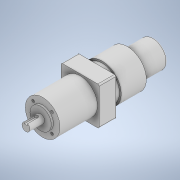
# Autodesk Inventor part: Motor
Saved by Autodesk Inventor 2020 (Build 240168000, 168)
## iProperties
Created: 2022-06-08
Part Number: Motor
Material: 일반
Document SubType Name: Modeling
Designer: samsung
Density: 1 g/cm^3
Appearance: 기본값
Mass: 368.156 g
Surface Area: 370.371 cm^2
Volume: 368.156 cm^3
Author: samsung
Autodesk Inventor part; units mm, degrees
ref_plane "YZ Plane" through (0, 0, 0) normal (1, 0, 0) x (0, 1, 0)
ref_plane "XZ Plane" through (0, 0, 0) normal (0, 1, 0) x (-1, 0, 0)
ref_plane "XY Plane" through (0, 0, 0) normal (0, 0, 1) x (1, 0, 0)
sketch "스케치1" plane through (0, 0, 0) normal (0, 0, 1) x (1, 0, 0)
  line L0 (-26.5, -28.5) -> (26.5, -28.5)
  line L1 (28.5, -26.5) -> (28.5, 26.5)
  line L2 (26.5, 28.5) -> (-26.5, 28.5)
  line L3 (-28.5, 26.5) -> (-28.5, -26.5)
  line L4 (-28.5, -28.5) -> (28.5, 28.5) construction
  line L5 (28.5, -28.5) -> (-28.5, 28.5) construction
  arc A0 (28.5, 26.5) -> (26.5, 28.5) centre (26.5, 26.5) ccw
  arc A1 (26.5, -28.5) -> (28.5, -26.5) centre (26.5, -26.5) ccw
  arc A2 (-28.5, -26.5) -> (-26.5, -28.5) centre (-26.5, -26.5) ccw
  arc A3 (-26.5, 28.5) -> (-28.5, 26.5) centre (-26.5, 26.5) ccw
  point P0 (0, 0)
  dimension "d0" = 57
  dimension "d1" = 57
  dimension "d2" = 2
  constraints: 12 end point, 8 point on circle, 8 point on line, 8 tangent, 4 centre point, 3 equal radius, 2 midpoint, 2 parallel, 1 horizontal, 1 perpendicular
  measures "d0" distance of L5.end L4.end
  measures "d1" distance of L4.end L5.start
  measures "d2" radius of A0
extrude "돌출1" add sketch "스케치1" along normal blind 25
sketch "스케치2" plane through (0, 0, 25) normal (0, 0, 1) x (1, 0, 0)
  circle A0 centre (0, 0) radius 26
  dimension "d5" = 52
  constraints: 1 centre point, 1 coincident
  measures "d5" diameter of A0
extrude "돌출2" add sketch "스케치2" along normal blind 56.1
sketch "스케치3" plane through (0, 0, 81.1) normal (0, 0, 1) x (1, 0, 0)
  circle A0 centre (0, 0) radius 16
  line L0 (0, 0) -> (20, 0) construction
  circle A1 centre (0, 0) radius 15
  point P0 (-14.1421, 14.1421)
  point P1 (-14.1421, -14.1421)
  point P2 (14.1421, -14.1421)
  point P3 (14.1421, 14.1421)
  dimension "d9" = 32
  dimension "d16" = 30
  constraints: 2 centre point, 2 end point, 1 coincident, 1 horizontal
  measures "d9" diameter of A0
  measures "d16" diameter of A1
sketch "스케치4" plane through (0, 0, 81.1) normal (0, 0, 1) x (1, 0, 0)
  circle A0 centre (0, 0) radius 16
  dimension "d21" = 32
  constraints: 1 centre point, 1 coincident
  measures "d21" diameter of A0
extrude "돌출5" add sketch "스케치4" along normal blind 3
sketch "스케치5" plane through (0, 0, 84.1) normal (0, 0, 1) x (1, 0, 0)
  circle A0 centre (0, 0) radius 6
  dimension "d24" = 12
  constraints: 1 centre point, 1 coincident
  measures "d24" diameter of A0
extrude "돌출6" add sketch "스케치5" along normal blind 22
sketch "스케치6" plane through (0, 0, 106.1) normal (0, 0, 1) x (1, 0, 0)
  circle A0 centre (0, 0) radius 6 projected
  circle A1 centre (0, 0) radius 6 projected
  line L0 (-2.5, 5.4544) -> (2.5, 5.4544)
  line L1 (2.5, 5.4544) -> (2.5, 2.9544)
  line L2 (2.5, 2.9544) -> (-2.5, 2.9544)
  line L3 (-2.5, 2.9544) -> (-2.5, 5.4544)
  line L4 (-2.5, 5.4544) -> (2.5, 5.4544)
  line L5 (2.5, 5.4544) -> (2.5, 6.5478)
  line L6 (2.5, 6.5478) -> (-2.5, 6.5478)
  line L7 (-2.5, 6.5478) -> (-2.5, 5.4544)
  dimension "d29" = 2.5
  constraints: 16 end point, 4 parallel, 2 horizontal, 2 perpendicular, 2 other
  measures "d29" distance of L0.end L1.end
extrude "돌출7" cut sketch "스케치6" against normal blind 15.5 contours L0 A0 | L1 L2 L3 L0 | A0 L7 L6 L5
sketch "스케치7" plane through (-2.5, 2.9544, 106.1) normal (0, 1, 0) x (1, 0, 0)
  line L0 (5, 0) -> (0, 0) projected
  line L1 (5, 0) -> (5, 15.5) projected
  line L2 (5, 15.5) -> (0, 15.5) projected
  line L3 (0, 0) -> (0, 15.5) projected
  circle A0 centre (2.5, 15.5) radius 2.5
  point P0 (2.5, 106.1)
  dimension "d32" = 5
  constraints: 1 centre point, 1 midpoint
  measures "d32" diameter of A0
extrude "돌출8" cut sketch "스케치7" along normal blind 15.5 contours A0 L2 | L2 A0
sketch "스케치8" plane through (0, 0, 0) normal (0, 0, -1) x (-1, 0, 0)
  circle A0 centre (0, 0) radius 28.5
  dimension "d35" = 57
  constraints: 1 centre point, 1 coincident
  measures "d35" diameter of A0
extrude "돌출9" add sketch "스케치8" along normal blind 45.8
sketch "스케치9" plane through (0, 0, -45.8) normal (0, 0, -1) x (-1, 0, 0)
  circle A0 centre (0, 0) radius 20
  dimension "d38" = 40
  constraints: 1 centre point, 1 coincident
  measures "d38" diameter of A0
extrude "돌출10" add sketch "스케치9" along normal blind 40
fillet "모깎기1" radius 2 1 edges at (20, 0, -85.8)
sketch "스케치10" plane through (0, 0, 0) normal (0, 0, -1) x (-1, 0, 0)
  point P0 (0, 0)
sketch "스케치11" plane through (0, 0, 0) normal (0, 0, -1) x (-1, 0, 0)
  circle A0 centre (0, 0) radius 26 projected
  line L0 (-28.5, -26.5) -> (-28.5, 26.5) projected
  arc A1 (-26.5, 28.5) -> (-28.5, 26.5) centre (-26.5, 26.5) ccw projected
  line L1 (-26.5, 28.5) -> (26.5, 28.5) projected
  arc A2 (28.5, 26.5) -> (26.5, 28.5) centre (26.5, 26.5) ccw projected
  line L2 (28.5, 26.5) -> (28.5, -26.5) projected
  arc A3 (26.5, -28.5) -> (28.5, -26.5) centre (26.5, -26.5) ccw projected
  line L3 (26.5, -28.5) -> (-26.5, -28.5) projected
  arc A4 (-28.5, -26.5) -> (-26.5, -28.5) centre (-26.5, -26.5) ccw projected
  circle A5 centre (0, 0) radius 26 projected
  circle A6 centre (22.4424, -22.4424) radius 2.5
  circle A7 centre (22.4424, 22.4424) radius 2.5
  circle A8 centre (-22.4424, 22.4424) radius 2.5
  circle A9 centre (-22.4424, -22.4424) radius 2.5
  dimension "d42" = 5
  dimension "d43" = 5
  dimension "d44" = 5
  dimension "d45" = 5
  constraints: 4 centre point
  measures "d42" diameter of A6
  measures "d43" diameter of A7
  measures "d44" diameter of A8
  measures "d45" diameter of A9
extrude "돌출11" add sketch "스케치11" along normal blind 3 contours A6 | A7 | A8 | A9
fillet "모깎기2" radius 1 4 edges at (-19.9424, 22.4424, -3) (-19.9424, -22.4424, -3) (24.9424, 22.4424, -3) (24.9424, -22.4424, -3)
sketch "스케치13" plane through (0, 0, 0) normal (0, 0, -1) x (-1, 0, 0)
  circle A0 centre (0, 0) radius 26 projected
  circle A1 centre (0, 0) radius 28.5
  dimension "d49" = 57
  constraints: 1 centre point, 1 coincident
  measures "d49" diameter of A1
extrude "돌출12" cut sketch "스케치13" along normal blind 8
hole "구멍1" at (-14.1421, 14.1421, 81.1) at (14.1421, 14.1421, 81.1) at (14.1421, -14.1421, 81.1) at (-14.1421, -14.1421, 81.1) direction (0, 0, -1) diameter 4.134 depth 10 tip angle 118 thread size "M5x0.8" class "6H" standard "ISO Metric profile"
